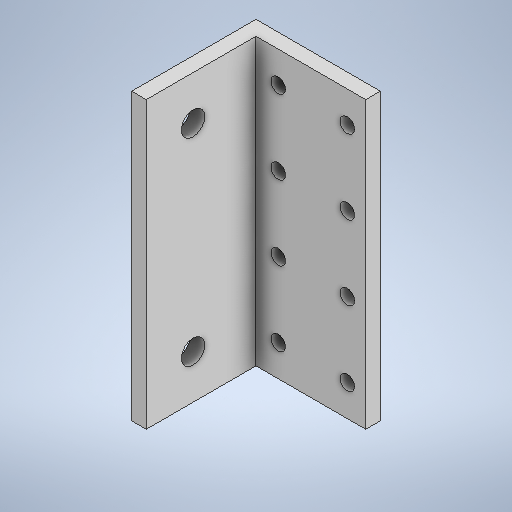
# Autodesk Inventor part: LongPluckMount
Saved by Autodesk Inventor 2025.1 (Build 291241000, 241)
## iProperties
Created: 2025-12-05
Part Number: LongPluckMount
Material: Generic
Document SubType Name: Modeling
Designer: Juxin
Density: 1 g/cm^3
Appearance: Default
Author: Juxin
Autodesk Inventor part; units mm, degrees
ref_plane "YZ Plane" through (0, 0, 0) normal (1, 0, 0) x (0, 1, 0)
ref_plane "XZ Plane" through (0, 0, 0) normal (0, 1, 0) x (-1, 0, 0)
ref_plane "XY Plane" through (0, 0, 0) normal (0, 0, 1) x (1, 0, 0)
sketch "Sketch1" plane through (0, 0, 0) normal (0, 1, 0) x (-1, 0, 0)
  line L0 (0, 0) -> (27.0002, 0)
  line L1 (27.0002, 0) -> (27.0002, -27.0002)
  line L2 (27.0002, -27.0002) -> (0, -27.0002)
  line L3 (0, -27.0002) -> (0, 0)
  line L4 (27.0002, -27.0002) -> (23.8252, -27.0002)
  line L5 (23.8252, -27.0002) -> (23.8252, -23.8252)
  line L6 (0, 0) -> (23.8252, 0)
  line L7 (23.8252, 0) -> (23.8252, -23.8252)
  line L8 (23.8252, -23.8252) -> (0, -23.8252)
  line L9 (0, -23.8252) -> (0, 0)
  dimension "d0" = 27.0002
  dimension "d1" = 27.0002
  dimension "d2" = 3.175
  dimension "d3" = 3.175
  dimension "d4" = 90
  constraints: 20 end point, 4 parallel, 3 perpendicular, 2 horizontal, 1 point on line
  measures "d0" distance of L1.end L2.end
  measures "d1" distance of L0.end L1.end
  measures "d2" distance of L1.end L4.end
  measures "d3" distance of L4.end L5.end
  measures "d4" angle of L4 L5
extrude "Extrusion1" add sketch "Sketch1" along normal blind 13.589 contours L0 L1 L2 L5 L7 | L8 L5 L2 L3
sketch "Sketch2" plane through (0, 0, -27.0002) normal (0, 0, -1) x (-1, 0, 0)
  line L0 (27.0002, 0) -> (27.0002, 13.589) projected
  line L1 (0, 0) -> (0, 13.589) projected
  line L2 (27.0002, 13.589) -> (0, 13.589)
  line L3 (0, 13.589) -> (0, 0)
  line L4 (0, 0) -> (27.0002, 0)
  line L5 (27.0002, 0) -> (27.0002, 13.589)
  line L6 (27.0002, 6.7945) -> (18.9992, 6.7945)
  circle A0 centre (18.9992, 6.7945) radius 1.5875
  line L7 (18.9992, 6.7945) -> (4.0132, 6.7945)
  line L8 (0, 0) -> (27.0002, 0) projected
  line L9 (18.9992, 6.7945) -> (33.9852, 6.7945) construction
  circle A1 centre (4.0132, 6.7945) radius 1.5875
  dimension "d7" = 13.589
  dimension "d8" = 8.001
  dimension "d9" = 3.175
  dimension "d10" = 14.986
  dimension "d11" = 180
  dimension "d12" = 3.175
  constraints: 14 end point, 3 horizontal, 3 parallel, 2 centre point, 2 coincident, 1 collinear, 1 midpoint, 1 perpendicular, 1 point on line
  measures "d7" distance of L3.end L2.end
  measures "d8" distance of L6.start L6.end
  measures "d9" diameter of A0
  measures "d10" distance of L7.start L7.end
  measures "d11" angle of L7 L9
  measures "d12" diameter of A1
extrude "Extrusion2" cut sketch "Sketch2" against normal blind 16.129 contours A0 L7 L6 | L6 L7 A0 | A1
move faces "Move1" translate (0, -16.129, 0) faces at (-16.9418, 0, -25.9419)
sketch "Sketch4" plane through (0, 13.589, -27.0002) normal (0, 0, -1) x (-1, 0, 0)
  line L0 (27.0002, -29.718) -> (27.0002, 0) projected
  line L1 (0, -29.718) -> (0, 0) projected
  line L2 (27.0002, -29.718) -> (0, -29.718)
  line L3 (0, -29.718) -> (0, -16.129)
  line L4 (0, -16.129) -> (27.0002, -16.129)
  line L5 (27.0002, -16.129) -> (27.0002, -29.718)
  line L6 (27.0002, -22.9235) -> (18.9992, -22.9235)
  line L7 (23.8252, -29.718) -> (23.8252, 0) projected
  line L8 (27.0002, -22.9235) -> (35.0012, -22.9235) construction
  circle A0 centre (18.9992, -22.9235) radius 1.5875
  line L9 (18.9992, -22.9235) -> (4.0132, -22.9235)
  circle A1 centre (4.0132, -22.9235) radius 1.5875
  point P0 (0, -13.589)
  dimension "d18" = 13.589
  dimension "d19" = 8.001
  dimension "d20" = 180
  dimension "d21" = 3.175
  dimension "d22" = 14.986
  dimension "d23" = 3.175
  constraints: 14 end point, 3 parallel, 2 centre point, 2 coincident, 2 horizontal, 2 perpendicular, 1 collinear, 1 midpoint, 1 point on line
  measures "d18" distance of L2.end L3.end
  measures "d19" distance of L6.start L6.end
  measures "d20" angle of L6 L8
  measures "d21" diameter of A0
  measures "d22" distance of L9.start L9.end
  measures "d23" diameter of A1
extrude "Extrusion3" cut sketch "Sketch4" against normal blind 13.589 contours A0 L9 L6 | L6 L9 A0 | A1
move faces "Move2" translate (0, -16.129, 0) faces at (-16.9418, -16.129, -25.9419)
sketch "Sketch5" plane through (0, 13.589, -27.0002) normal (0, 0, -1) x (-1, 0, 0)
  line L0 (0, -45.847) -> (27.0002, -45.847) projected
  line L1 (0, -45.847) -> (0, 0) projected
  line L2 (27.0002, -45.847) -> (0, -45.847)
  line L3 (0, -45.847) -> (0, -32.258)
  line L4 (0, -32.258) -> (27.0002, -32.258)
  line L5 (27.0002, -32.258) -> (27.0002, -45.847)
  line L6 (27.0002, -45.847) -> (27.0002, 0) projected
  line L7 (27.0002, -39.0525) -> (18.9992, -39.0525)
  circle A0 centre (18.9992, -39.0525) radius 1.5875
  line L8 (18.9992, -39.0525) -> (4.0132, -39.0525)
  circle A1 centre (4.0132, -39.0525) radius 1.5875
  point P0 (0, -13.589)
  dimension "d29" = 13.589
  dimension "d31" = 8.001
  dimension "d32" = 3.175
  dimension "d33" = 14.986
  dimension "d34" = 3.175
  constraints: 12 end point, 2 centre point, 2 coincident, 2 horizontal, 2 parallel, 2 perpendicular, 2 point on line
  measures "d29" distance of L2.end L3.end
  measures "d31" distance of L7.start L7.end
  measures "d32" diameter of A0
  measures "d33" distance of L8.start L8.end
  measures "d34" diameter of A1
extrude "Extrusion4" cut sketch "Sketch5" against normal blind 13.589 contours A0 L8 L7 | L7 L8 A0 | A1
move faces "Move3" translate (0, -16.129, 0) faces at (-16.9418, -32.258, -25.9419)
sketch "Sketch6" plane through (0, 13.589, -27.0002) normal (0, 0, -1) x (-1, 0, 0)
  line L0 (27.0002, -61.976) -> (27.0002, 0) projected
  line L1 (0, -61.976) -> (0, 0) projected
  line L2 (27.0002, -61.976) -> (0, -61.976)
  line L3 (0, -61.976) -> (0, -48.387)
  line L4 (0, -48.387) -> (27.0002, -48.387)
  line L5 (27.0002, -48.387) -> (27.0002, -61.976)
  line L6 (27.0002, -55.1815) -> (18.9992, -55.1815)
  circle A0 centre (18.9992, -55.1815) radius 1.5875
  line L7 (18.9992, -55.1815) -> (4.0132, -55.1815)
  line L8 (18.9992, -55.1815) -> (33.9852, -55.1815) construction
  circle A1 centre (4.0132, -55.1815) radius 1.5875
  point P0 (0, -13.589)
  dimension "d40" = 13.589
  dimension "d41" = 8.001
  dimension "d42" = 3.175
  dimension "d43" = 14.986
  dimension "d44" = 180
  dimension "d45" = 3.175
  constraints: 14 end point, 4 horizontal, 2 centre point, 2 coincident, 2 parallel, 1 collinear, 1 midpoint, 1 perpendicular, 1 point on line
  measures "d40" distance of L2.end L3.end
  measures "d41" distance of L6.start L6.end
  measures "d42" diameter of A0
  measures "d43" distance of L7.start L7.end
  measures "d44" angle of L7 L8
  measures "d45" diameter of A1
extrude "Extrusion5" cut sketch "Sketch6" against normal blind 13.589 contours A0 L7 L6 | L6 L7 A0 | A1
sketch "Sketch7" plane through (-27.0002, 13.589, -27.0002) normal (-1, 0, 0) x (0, 0, 1)
  line L0 (27.0002, -61.976) -> (27.0002, 0) projected
  line L1 (27.0002, -61.976) -> (16.8402, -61.976)
  line L2 (0, -61.976) -> (27.0002, -61.976) projected
  line L3 (16.8402, -61.976) -> (16.8402, -52.451)
  line L4 (27.0002, 0) -> (3.175, 0) projected
  line L5 (27.0002, 0) -> (16.8402, 0)
  line L6 (16.8402, 0) -> (16.8402, -9.525)
  circle A0 centre (16.8402, -9.525) radius 2.54
  circle A1 centre (16.8402, -52.451) radius 2.54
  point P0 (27.0002, -13.589)
  dimension "d48" = 10.16
  dimension "d49" = 9.525
  dimension "d50" = 90
  dimension "d51" = 10.16
  dimension "d52" = 9.525
  dimension "d53" = 270
  dimension "d54" = 5.08
  dimension "d55" = 5.08
  constraints: 8 end point, 2 centre point, 2 coincident, 2 perpendicular, 2 point on line
  measures "d48" distance of L0.start L1.end
  measures "d49" distance of L1.end L3.end
  measures "d50" angle of L1 L3
  measures "d51" distance of L0.end L5.end
  measures "d52" distance of L5.end L6.end
  measures "d54" diameter of A0
  measures "d55" diameter of A1
extrude "Extrusion6" cut sketch "Sketch7" against normal blind 13.589
body "Solid1"
